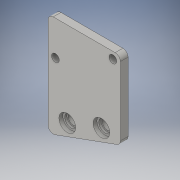
# Autodesk Inventor part: bump_switch_mount
Saved by Autodesk Inventor 2016 (Build 200138000, 138)
## iProperties
Created: 2016-02-16
Part Number: bump_switch_mount
Material: Generic
Document SubType Name: Modeling
Designer: jforce
Density: 1 g/cm^3
Appearance: Default
Author: jforce
Autodesk Inventor part; units mm, degrees
ref_plane "YZ Plane" through (0, 0, 0) normal (1, 0, 0) x (0, 1, 0)
ref_plane "XZ Plane" through (0, 0, 0) normal (0, 1, 0) x (-1, 0, 0)
ref_plane "XY Plane" through (0, 0, 0) normal (0, 0, 1) x (1, 0, 0)
sketch "Sketch1" plane through (0, 0, 0) normal (0, 0, 1) x (1, 0, 0)
  line L0 (0, 61.5875) -> (62, 61.5875) construction
  line L1 (62, 61.5875) -> (62, -0.4125) construction
  line L2 (62, -0.4125) -> (0, -0.4125) construction
  line L3 (0, -0.4125) -> (0, 61.5875) construction
  line L4 (48.4322, 11.2012) -> (48.4322, 37.9079)
  line L5 (20.3147, 37.9079) -> (20.3147, 2.4417)
  line L6 (24.0433, 39.9079) -> (22.3147, 39.9079)
  line L7 (46.4322, 39.9079) -> (24.0433, 39.9079)
  arc A0 (22.3147, 39.9079) -> (20.3147, 37.9079) centre (22.3147, 37.9079) ccw
  circle A1 centre (23.179, 26.4983) radius 1.5
  circle A2 centre (45.5157, 37.2749) radius 1.5
  line L8 (16.613, -7.1773) -> (55.7088, 13.6823) projected
  line L9 (22.9974, 0.5619) -> (47.1149, 9.3214)
  arc A3 (20.3147, 2.4417) -> (22.9974, 0.5619) centre (22.3147, 2.4417) ccw
  arc A4 (47.1149, 9.3214) -> (48.4322, 11.2012) centre (46.4322, 11.2012) ccw
  arc A5 (48.4322, 37.9079) -> (46.4322, 39.9079) centre (46.4322, 37.9079) ccw
  point P0 (0, 0)
  point P1 (48.4322, 39.9079)
  point P2 (48.4322, 9.7998)
  point P3 (20.3147, -0.4125)
  dimension "d9" = 62
  dimension "d18" = 2
  dimension "d19" = 3
  dimension "d20" = 3
  dimension "d27" = 28.1175
  dimension "d47" = 2
  constraints: 10 end point, 8 point on circle, 8 point on line, 8 tangent, 6 centre point, 2 equal radius, 1 parallel, 2 other
  measures "d9" distance between parallel lines of L1 L3
  measures "d18" radius of A0
  measures "d19" diameter of A1
  measures "d20" diameter of A2
  measures "d27" distance between parallel lines of L4 L5
  measures "d47" radius of A3
extrude "Extrusion2" add sketch "Sketch1" along normal blind 3
sketch "Sketch3" plane through (0, 0, 0) normal (0, 0, -1) x (-1, 0, 0)
  circle A0 centre (-41.0584, 11.8538) radius 4
  circle A1 centre (-27.789, 6.9341) radius 4
  point P0 (0, 0)
  dimension "d51" = 8
  dimension "d52" = 8
  constraints: 2 centre point
  measures "d51" diameter of A0
  measures "d52" diameter of A1
extrude "Extrusion4" add sketch "Sketch3" along normal blind 1.5
sketch "Sketch4" plane through (0, 0, 3) normal (0, 0, 1) x (1, 0, 0)
  circle A0 centre (27.789, 6.9341) radius 4 projected
  circle A1 centre (41.0584, 11.8538) radius 4 projected
  circle A2 centre (41.0584, 11.8538) radius 3.25
  circle A3 centre (27.789, 6.9341) radius 3.25
  point P0 (0, 0)
  dimension "d55" = 6.5
  dimension "d56" = 6.5
  constraints: 2 centre point, 2 coincident
  measures "d55" diameter of A2
  measures "d56" diameter of A3
extrude "Extrusion5" cut sketch "Sketch4" against normal blind 1.5 contours A2 | A3
sketch "Sketch5" plane through (41.0584, 11.8538, 1.5) normal (0, 0, 1) x (1, 0, 0)
  circle A0 centre (-13.2694, -4.9197) radius 3.25 projected
  circle A1 centre (0, 0) radius 3.25 projected
  point P0 (-41.0584, -11.8538)
hole "Hole1" at (27.789, 6.9341, 1.5) at (41.0584, 11.8538, 1.5) direction (0, 0, -1) diameter 4 depth 3 tip angle 118 counterbore diameter 5 counterbore depth 0.85
body "Solid2"
